WingedNutThroughScrewDouble3mm_v4 (Autodesk Fusion 360 design; units mm, degrees)
Autodesk Fusion 360 part; units mm, degrees
sketch "Sketch1" plane through (0, 0, 0) normal (0, 0, 1) x (1, 0, 0)
  circle A0 centre (0, 0) radius 1.1
  line L0 (1.1836, -2.05) -> (2.3671, 0)
  line L1 (2.3671, 0) -> (1.1836, 2.05)
  line L2 (1.1836, 2.05) -> (-1.1836, 2.05)
  line L3 (-1.1836, 2.05) -> (-2.3671, 0)
  line L4 (-2.3671, 0) -> (-1.1836, -2.05)
  line L5 (-1.1836, -2.05) -> (1.1836, -2.05)
  circle A1 centre (-6, 0) radius 1.5
  circle A2 centre (-5.3127, -2.7883) radius 1.5
  circle A3 centre (-3.4084, -4.9379) radius 1.5
  circle A4 centre (-0.7232, -5.9563) radius 1.5
  circle A5 centre (2.1276, -5.6101) radius 1.5
  circle A6 centre (4.4911, -3.9787) radius 1.5
  circle A7 centre (5.8257, -1.4359) radius 1.5
  circle A8 centre (5.8257, 1.4359) radius 1.5
  circle A9 centre (4.4911, 3.9787) radius 1.5
  circle A10 centre (2.1276, 5.6101) radius 1.5
  circle A11 centre (-0.7232, 5.9563) radius 1.5
  circle A12 centre (-3.4084, 4.9379) radius 1.5
  circle A13 centre (-5.3127, 2.7883) radius 1.5
  circle A14 centre (-4.5, 0.0086) radius 1
  circle A15 centre (-0.0086, -4.5) radius 1
  circle A16 centre (4.5, -0.0086) radius 1
  circle A17 centre (0.0086, 4.5) radius 1
  circle A18 centre (29.8257, 1.4359) radius 1.5
  circle A19 centre (18.6873, 2.7883) radius 1.5
  circle A20 centre (20.5916, 4.9379) radius 1.5
  circle A21 centre (20.5916, -4.9379) radius 1.5
  circle A22 centre (28.4911, 3.9787) radius 1.5
  line L6 (22.8164, 2.04) -> (21.6329, -0.01)
  circle A23 centre (26.1276, 5.6101) radius 1.5
  circle A24 centre (26.1276, -5.6101) radius 1.5
  circle A25 centre (18, 0) radius 1.5
  circle A26 centre (28.5, -0.0086) radius 1
  line L7 (22.8164, -2.06) -> (25.1836, -2.06)
  circle A27 centre (23.2768, -5.9563) radius 1.5
  line L8 (25.1836, 2.04) -> (22.8164, 2.04)
  circle A28 centre (19.5, 0.0086) radius 1
  circle A29 centre (29.8257, -1.4359) radius 1.5
  circle A30 centre (23.9914, -4.5) radius 1
  circle A31 centre (24.0086, 4.5) radius 1
  circle A32 centre (18.6873, -2.7883) radius 1.5
  circle A33 centre (24, 0) radius 1.1
  circle A34 centre (28.4911, -3.9787) radius 1.5
  circle A35 centre (23.2768, 5.9563) radius 1.5
  line L9 (21.6329, -0.01) -> (22.8164, -2.06)
  line L10 (25.1836, -2.06) -> (26.3671, -0.01)
  line L11 (26.3671, -0.01) -> (25.1836, 2.04)
  point P0 (24, 0)
  point P1 (24, -0.01)
  dimension "d6" = 2.2
  dimension "d8" = 3
  dimension "d10" = 6
  dimension "d12" = 360
  dimension "d33" = 2
  dimension "d36" = 4.5
  dimension "d45" = 2.2
  dimension "d47" = 3
  dimension "d48" = 6
  dimension "d50" = 4.5
  dimension "d55" = 4.1
  dimension "d56" = 4.1
  constraint coincident A0.centre origin
  constraint equal A14 A17
  constraint equal A16 A17
  constraint equal A15 A16
  constraint equal A15 A31
  constraint equal A28 A31
  constraint equal A28 A30
  constraint equal A26 A30
  measures "d6" diameter of A0
  measures "d8" diameter of A1
  measures "d10" distance of A0.centre A1.centre
  measures "d33" diameter of A14
  measures "d36" horizontal distance of A0.centre A14.centre
  measures "d45" diameter of A33
  measures "d47" diameter of A25
  measures "d48" distance of A25.centre P0
  measures "d50" horizontal distance of A28.centre P0
  measures "d55" distance of L2 L5
  measures "d56" distance of L7 L8
extrude "Extrude1" add sketch "Sketch1" along normal blind 3.1 contours A0 | L0 L1 L2 L3 L4 L5 | A1 A14 | A1 A14 | A1 A2 A13 A14 | A1 A2 A3 A4 A5 A6 A7 A8 A9 A10 A11 A12 A13 A14 A15 A16 A17 | A1 A13 | A1 A12 A13 | A1 A2 A3 | A1 A2 | A12 A13 | A11 A12 A13 | A2 A3 | A2 A3 A4 | A11 A12 | A10 A11 A12 A17 | A3 A4 | A3 A4 A5 A15 | A10 A11 | A9 A10 A11 A17 | A4 A5 | A4 A5 A6 A15 | A10 A11 A17 | A11 A17 | A10 A11 A17 | A4 A5 A15 | A4 A15 | A4 A5 A15 | A9 A10 | A8 A9 A10 | A10 A17 | A5 A15 | A5 A6 | A5 A6 A7 | A8 A9 | A7 A8 A9 A16 | A6 A7 A8 A16 | A6 A7 | A7 A8 A16 | A7 A8 A16 | A7 A8 A16 | A7 A8 A16 | A7 A8 A16 makes body 1
extrude "Extrude2" cut sketch "Sketch1" along normal blind 3.1 contours A0 bodies 1
extrude "Extrude3" cut sketch "Sketch1" along normal blind 1.6 from surface at 1.5 contours L0 L1 L2 L3 L4 L5 bodies 1
copy_body "CopyPasteBodies2" bodies 1 makes body 2
move_body "Move2" bodies 2 to x (1, 0, 0) y (0, 1, 0) z (0, 0, 1) at (24, 0, 0)
extrude "Extrude5" add sketch "Sketch1" along normal blind 6.2 draft -2 contours A1 A14 | A1 A14 | A11 A17 | A10 A11 A17 | A4 A5 A15 | A4 A15 | A10 A17 | A5 A15 | A7 A8 A16 | A7 A8 A16 | A7 A8 A16 | A7 A8 A16 picked at (0.7033, 4.6344) picked at (0.6844, -4.7015) picked at (4.8814, 0.5124) picked at (4.2975, -0.0045) picked at (4.8982, -0.5054) picked at (5.4756, 0.0012) bodies 1
extrude "Extrude6" cut sketch "Sketch1" along normal blind 6.2 contours A18 A26 A29 | A18 A26 A29 | A18 A26 A29 | A18 A26 A29 | A23 A31 A35 | A23 A31 | A31 A35 | A24 A30 | A24 A27 A30 | A27 A30 | A25 A28 | A25 A28 picked at (28.8982, -0.5054) picked at (29.4756, 0.0012) picked at (28.8814, 0.5124) picked at (28.2975, -0.0045) picked at (24.7033, 4.6344) picked at (24.6844, -4.7015) bodies 2
fillet "Fillet3" radius 0.4 4 edges at (-5.2305, 0.292, 6.2) (-0.7391, -4.2167, 6.2) (-0.7218, 4.7833, 6.2) (3.7695, 0.2747, 6.2) on bodies 1
equation "screwDiam = 2.2 mm"
equation "FlatSideNutDistance = 4.1 mm"
equation "solidBaseHeight = 1.5 mm"
equation "nutHeight = 1.6 mm"
equation "wingDiameter = 12 mm"
equation "d6 = screwDiam"
equation "d10 = wingDiameter / 2"
equation "d11 = bumpCicles"
equation "d12 = 360.00 °"
equation "bumpCicles = 13"
equation "d14 = nutHeight + solidBaseHeight"
equation "d16 = nutHeight + solidBaseHeight"
equation "d18 = solidBaseHeight"
equation "d19 = nutHeight"
equation "d36 = wingDiameter / 2 - 1.5 mm"
equation "d41 = ( nutHeight + solidBaseHeight ) * 2"
equation "d45 = screwDiam"
equation "d48 = wingDiameter / 2"
equation "d50 = wingDiameter / 2 - 1.5 mm"
equation "d51 = ( nutHeight + solidBaseHeight ) * 2"
equation "d55 = FlatSideNutDistance"
equation "d56 = FlatSideNutDistance"
named bodies: "wing", "wing (1)"
